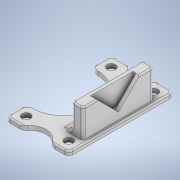
# Autodesk Inventor part: syringe pump holder
Saved by Autodesk Inventor 2021 (Build 250183000, 183)
## iProperties
Created: 2020-11-04
Part Number: syringe pump holder
Material: Generic
Document SubType Name: Modeling
Designer: User01
Density: 1 g/cm^3
Appearance: Default
Author: User01
Autodesk Inventor part; units mm, degrees
ref_plane "YZ Plane" through (0, 0, 0) normal (1, 0, 0) x (0, 1, 0)
ref_plane "XZ Plane" through (0, 0, 0) normal (0, 1, 0) x (-1, 0, 0)
sketch "Sketch1" plane through (0, 0, 0) normal (0, 1, 0) x (-1, 0, 0)
  circle A0 centre (-1.6554, 3.0337) radius 3
  circle A1 centre (-1.6554, -56.9663) radius 3
  circle A2 centre (-31.6554, -56.9663) radius 3
  circle A3 centre (-31.6554, 3.0337) radius 3
  line L0 (5.3446, 10.0337) -> (-38.6554, 10.0337)
  line L1 (-38.6554, 10.0337) -> (-38.6554, -63.9663)
  line L2 (-38.6554, -63.9663) -> (5.3446, -63.9663)
  line L3 (5.3446, -63.9663) -> (5.3446, 10.0337)
  line L4 (9.976, -3.9663) -> (-45.5967, -3.9663) construction
  line L5 (12.0147, -49.9663) -> (-48.9508, -49.9663) construction
  line L6 (-6.6554, 28.7025) -> (-6.6554, -79.6712) construction
  line L7 (-26.6554, 36.5804) -> (-26.6554, -80.7358) construction
  line L8 (10.9665, 4.0337) -> (-48.9508, 4.0337) construction
  arc A4 (-26.6554, 10.0337) -> (-6.6554, 10.0337) centre (-16.6554, 15.367) ccw
  line L9 (7.2178, -57.9663) -> (-47.3026, -57.9663) construction
  arc A5 (-6.6554, -63.9663) -> (-26.6554, -63.9663) centre (-16.6554, -69.2997) ccw
  line L10 (5.3446, -3.9663) -> (-21.6554, -3.9663)
  line L11 (-21.6554, -3.9663) -> (-21.6554, -49.9663)
  line L12 (-21.6554, -49.9663) -> (5.3446, -49.9663)
  line L13 (5.3446, -49.9663) -> (5.3446, -3.9663)
  point P0 (0, 0)
  point P1 (5.3446, -49.9663)
  point P2 (-38.6554, -49.9663)
  point P3 (-38.6554, -3.9663)
  point P4 (5.3446, -49.9663)
  dimension "d0" = 6
  dimension "d1" = 6
  dimension "d2" = 6
  dimension "d3" = 6
  dimension "d4" = 36
  dimension "d5" = 66
  dimension "d7" = 4
  dimension "d8" = 66
  dimension "d9" = 4
  dimension "d10" = 4
  dimension "d11" = 4
  dimension "d52" = 12
  dimension "d53" = 12
  dimension "d54" = 14
  dimension "d55" = 6
  dimension "d56" = 6
  dimension "d62" = 5
  constraints: 28 end point, 17 point on line, 6 centre point, 6 horizontal, 4 parallel, 4 point on circle, 4 vertical, 2 perpendicular, 2 tangent
  measures "d0" diameter of A0
  measures "d1" diameter of A1
  measures "d2" diameter of A2
  measures "d3" diameter of A3
  measures "d7" distance edge to line of A0 L3
  measures "d9" distance edge to line of A0 L0
  measures "d10" distance edge to line of A1 L2
  measures "d11" distance edge to line of A3 L1
  measures "d52" distance between parallel lines of L3 L6
  measures "d53" distance between parallel lines of L1 L7
  measures "d54" distance between parallel lines of L0 L4
  measures "d55" distance between parallel lines of L0 L8
  measures "d56" distance between parallel lines of L2 L9
  measures "d62" distance between parallel lines of L7 L11
extrude "Extrusion1" add sketch "Sketch1" along normal blind 3 contours L3 L10 L11 L12 L2 A5 L1 L0 A4
sketch "Sketch2" plane through (0, 3, 0) normal (0, 1, 0) x (1, 0, 0)
  line L0 (36.6554, 1.9663) -> (36.6554, 51.9663)
  line L1 (28.6554, 1.9663) -> (28.6554, 51.9663)
  line L2 (-5.3446, 26.9663) -> (46.0803, 26.9663) construction
  line L3 (28.6554, 1.9663) -> (36.6554, 1.9663)
  line L4 (28.6554, 51.9663) -> (36.6554, 51.9663)
  line L5 (38.6554, -10.0337) -> (38.6554, 63.9663) projected
  point P0 (0, 0)
  dimension "d20" = 25
  dimension "d21" = 25
  dimension "d59" = 8
  dimension "d60" = 2
  constraints: 10 end point, 3 horizontal, 1 perpendicular
  measures "d20" distance between parallel lines of L2 L3
  measures "d21" distance between parallel lines of L4 L2
  measures "d59" distance between parallel lines of L1 L0
  measures "d60" distance between parallel lines of L5 L0
extrude "Extrusion2" add sketch "Sketch2" along normal blind 20
ref_plane "Work Plane1" through (34.1554, 3, -1.9663) normal (1, 0, 0) x (0, 0, -1)
sketch "Sketch3" plane through (34.1554, 3, -1.9663) normal (1, 0, 0) x (0, 0, -1)
  line L0 (0, 20) -> (50, 20) projected
  line L1 (25, 20) -> (10, 20)
  line L2 (10, 20) -> (10, 5)
  line L3 (10, 5) -> (25, 5)
  line L4 (25, 20) -> (40, 20)
  line L5 (40, 20) -> (40, 5)
  line L6 (40, 5) -> (25, 5)
  line L7 (10, 20) -> (25, 5)
  line L8 (40, 20) -> (25, 5)
  point P0 (-1.9663, -3)
  dimension "d23" = 15
  dimension "d24" = 15
  dimension "d25" = 15
  dimension "d26" = 15
  constraints: 16 end point, 2 horizontal, 2 parallel, 2 perpendicular, 1 midpoint
  measures "d23" distance of L3.end L2.end
  measures "d24" distance of L2.end L1.end
  measures "d25" distance of L5.end L6.end
  measures "d26" distance of L4.end L5.end
extrude "Extrusion3" cut sketch "Sketch3" along normal blind 2.5 contours L0 L8 L7
sketch "Sketch4" plane through (0, 23, 0) normal (0, 1, 0) x (1, 0, 0)
  line L0 (34.1554, 11.9663) -> (34.1554, 26.9663) projected
  line L1 (34.1554, 11.9663) -> (31.9554, 11.9663)
  line L2 (31.9554, 11.9663) -> (31.9554, 41.9663)
  line L3 (31.9554, 41.9663) -> (34.1554, 41.9663)
  line L4 (34.1554, 41.9663) -> (34.1554, 11.9663)
  line L5 (34.1554, 26.9663) -> (36.6554, 26.9663) projected
  point P0 (0, 0)
  dimension "d29" = 2.2
  dimension "d31" = 15
  dimension "d32" = 15
  constraints: 8 end point, 2 parallel, 1 horizontal, 1 perpendicular, 1 point on line
  measures "d29" distance of L2.end L3.end
  measures "d31" distance between parallel lines of L5 L1
  measures "d32" distance between parallel lines of L5 L3
extrude "Extrusion4" cut sketch "Sketch4" against normal blind 15
fillet "Fillet1" radius 1 12 edges at (38.6554, 3, -26.9663) (0.6554, 3, -63.9663) (32.6554, 3, -63.9663) (-5.3446, 3, 3.0337) (-5.3446, 3, -56.9663) (0.6554, 3, 10.0337) (32.6554, 3, 10.0337) (28.6554, 23, -26.9663) (32.6554, 23, -1.9663) (36.6554, 23, -6.9663) (36.6554, 23, -46.9663) (32.6554, 23, -51.9663)
fillet "Fillet1" radius 3 4 edges at (-5.3446, 1.5, -63.9663) (38.6554, 1.5, -63.9663) (38.6554, 1.5, 10.0337) (-5.3446, 1.5, 10.0337)
fillet "Fillet1" radius 5 6 edges at (6.6554, 1.5, -63.9663) (26.6554, 1.5, -63.9663) (-5.3446, 1.5, -3.9663) (6.6554, 1.5, 10.0337) (26.6554, 1.5, 10.0337) (-5.3446, 1.5, -49.9663)
fillet "Fillet1" radius 23 2 edges at (21.6554, 1.5, -49.9663) (21.6554, 1.5, -3.9663)
fillet "Fillet1" radius 7 1 edges at (28.6554, 3, -26.9663)
fillet "Fillet1" radius 2 4 edges at (36.6554, 13, -1.9663) (28.6554, 13, -1.9663) (28.6554, 13, -51.9663) (36.6554, 13, -51.9663)
sketch "Sketch5" plane through (31.9554, 8, -11.9663) normal (1, 0, 0) x (0, 0, -1)
  line L0 (0, 15) -> (0, 0) projected
  line L1 (0, 14) -> (1, 14)
  line L2 (1, 0) -> (0, 0)
  line L3 (0, 0) -> (0, 14)
  line L4 (0, 14) -> (30, 14) projected
  line L5 (1, 14) -> (1, 0)
  line L6 (1, 14) -> (2, 14)
  line L7 (2, 0) -> (1, 0)
  line L8 (1, 0) -> (1, 14)
  line L9 (2, 14) -> (2, 0)
  line L10 (2, 14) -> (3, 14)
  line L11 (3, 0) -> (2, 0)
  line L12 (2, 0) -> (2, 14)
  line L13 (3, 14) -> (3, 0)
  line L14 (3, 14) -> (4, 14)
  line L15 (4, 0) -> (3, 0)
  line L16 (3, 0) -> (3, 14)
  line L17 (4, 14) -> (4, 0)
  line L18 (4, 14) -> (5, 14)
  line L19 (5, 0) -> (4, 0)
  line L20 (4, 0) -> (4, 14)
  line L21 (5, 14) -> (5, 0)
  line L22 (5, 14) -> (6, 14)
  line L23 (6, 0) -> (5, 0)
  line L24 (5, 0) -> (5, 14)
  line L25 (6, 14) -> (6, 0)
  line L26 (6, 14) -> (7, 14)
  line L27 (7, 0) -> (6, 0)
  line L28 (6, 0) -> (6, 14)
  line L29 (7, 14) -> (7, 0)
  line L30 (7, 14) -> (8, 14)
  line L31 (8, 0) -> (7, 0)
  line L32 (7, 0) -> (7, 14)
  line L33 (8, 14) -> (8, 0)
  line L34 (8, 14) -> (9, 14)
  line L35 (9, 0) -> (8, 0)
  line L36 (8, 0) -> (8, 14)
  line L37 (9, 14) -> (9, 0)
  line L38 (9, 14) -> (10, 14)
  line L39 (10, 0) -> (9, 0)
  line L40 (9, 0) -> (9, 14)
  line L41 (10, 14) -> (10, 0)
  line L42 (10, 14) -> (11, 14)
  line L43 (11, 0) -> (10, 0)
  line L44 (10, 0) -> (10, 14)
  line L45 (11, 14) -> (11, 0)
  line L46 (11, 14) -> (12, 14)
  line L47 (12, 0) -> (11, 0)
  line L48 (11, 0) -> (11, 14)
  line L49 (12, 14) -> (12, 0)
  line L50 (12, 14) -> (13, 14)
  line L51 (13, 0) -> (12, 0)
  line L52 (12, 0) -> (12, 14)
  line L53 (13, 14) -> (13, 0)
  line L54 (13, 14) -> (14, 14)
  line L55 (14, 0) -> (13, 0)
  line L56 (13, 0) -> (13, 14)
  line L57 (14, 14) -> (14, 0)
  line L58 (14, 14) -> (15, 14)
  line L59 (15, 0) -> (14, 0)
  line L60 (14, 0) -> (14, 14)
  line L61 (15, 14) -> (15, 0)
  line L62 (15, 14) -> (16, 14)
  line L63 (16, 0) -> (15, 0)
  line L64 (15, 0) -> (15, 14)
  line L65 (16, 14) -> (16, 0)
  line L66 (16, 14) -> (17, 14)
  line L67 (17, 0) -> (16, 0)
  line L68 (16, 0) -> (16, 14)
  line L69 (17, 14) -> (17, 0)
  line L70 (17, 14) -> (18, 14)
  line L71 (18, 0) -> (17, 0)
  line L72 (17, 0) -> (17, 14)
  line L73 (18, 14) -> (18, 0)
  line L74 (18, 14) -> (19, 14)
  line L75 (19, 0) -> (18, 0)
  line L76 (18, 0) -> (18, 14)
  line L77 (19, 14) -> (19, 0)
  line L78 (19, 14) -> (20, 14)
  line L79 (20, 0) -> (19, 0)
  line L80 (19, 0) -> (19, 14)
  line L81 (20, 14) -> (20, 0)
  line L82 (20, 14) -> (21, 14)
  line L83 (21, 0) -> (20, 0)
  line L84 (20, 0) -> (20, 14)
  line L85 (21, 14) -> (21, 0)
  line L86 (21, 14) -> (22, 14)
  line L87 (22, 0) -> (21, 0)
  line L88 (21, 0) -> (21, 14)
  line L89 (22, 14) -> (22, 0)
  line L90 (22, 14) -> (23, 14)
  line L91 (23, 0) -> (22, 0)
  line L92 (22, 0) -> (22, 14)
  line L93 (23, 14) -> (23, 0)
  line L94 (23, 14) -> (24, 14)
  line L95 (24, 0) -> (23, 0)
  line L96 (23, 0) -> (23, 14)
  line L97 (24, 14) -> (24, 0)
  line L98 (24, 14) -> (25, 14)
  line L99 (25, 0) -> (24, 0)
  line L100 (24, 0) -> (24, 14)
  line L101 (25, 14) -> (25, 0)
  line L102 (25, 14) -> (26, 14)
  line L103 (26, 0) -> (25, 0)
  line L104 (25, 0) -> (25, 14)
  line L105 (26, 14) -> (26, 0)
  line L106 (26, 14) -> (27, 14)
  line L107 (27, 0) -> (26, 0)
  line L108 (26, 0) -> (26, 14)
  line L109 (27, 14) -> (27, 0)
  line L110 (27, 14) -> (28, 14)
  line L111 (28, 0) -> (27, 0)
  line L112 (27, 0) -> (27, 14)
  line L113 (28, 14) -> (28, 0)
  line L114 (28, 14) -> (29, 14)
  line L115 (29, 0) -> (28, 0)
  line L116 (28, 0) -> (28, 14)
  line L117 (29, 14) -> (29, 0)
  line L118 (29, 14) -> (30, 14)
  line L119 (30, 0) -> (29, 0)
  line L120 (29, 0) -> (29, 14)
  line L121 (30, 14) -> (30, 0)
  point P0 (-11.9663, -8)
  point P1 (30, 0)
  point P2 (29, 14)
  point P3 (19, 14)
  point P4 (16, 14)
  point P5 (14, 0)
  point P6 (14, 14)
  point P7 (12, 0)
  point P8 (13, 14)
  point P9 (11, 14)
  point P10 (8, 0)
  point P11 (8, 14)
  point P12 (7, 14)
  point P13 (5, 14)
  point P14 (4, 14)
  point P15 (2, 0)
  point P16 (3, 14)
  dimension "d37" = 1
  dimension "d40" = 1
  constraints: 240 end point, 116 horizontal alignment, 59 parallel, 58 collinear, 1 horizontal, 1 perpendicular, 2 other
  measures "d37" distance between parallel lines of L3 L5
  measures "d40" distance of L2.end L7.end
body "Solid1"
